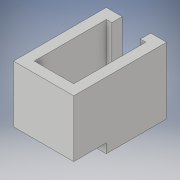
# Autodesk Inventor part: servo housing
Saved by Autodesk Inventor 2017 (Build 210142000, 142)
## iProperties
Created: 2017-01-19
Part Number: servo housing
Material: Generic
Document SubType Name: Modeling
Designer: Gabe Madonna
Density: 1 g/cm^3
Appearance: Default
Author: Gabe Madonna
Autodesk Inventor part; units mm, degrees
ref_plane "YZ Plane" through (0, 0, 0) normal (1, 0, 0) x (0, 1, 0)
ref_plane "XZ Plane" through (0, 0, 0) normal (0, 1, 0) x (-1, 0, 0)
ref_plane "XY Plane" through (0, 0, 0) normal (0, 0, 1) x (1, 0, 0)
sketch "Sketch1" plane through (0, 0, 0) normal (0, 1, 0) x (-1, 0, 0)
  line L0 (6.225, 11.375) -> (-6.225, 11.375)
  line L1 (-6.225, 11.375) -> (-6.225, -11.375)
  line L2 (-6.225, -11.375) -> (6.225, -11.375)
  line L3 (6.225, -11.375) -> (6.225, 11.375)
  line L4 (6.225, 11.375) -> (-6.225, -11.375) construction
  line L5 (-6.225, 11.375) -> (6.225, -11.375) construction
  line L6 (9.525, 14.675) -> (-9.525, 14.675)
  line L7 (-9.525, 14.675) -> (-9.525, -14.675)
  line L8 (-9.525, -14.675) -> (9.525, -14.675)
  line L9 (9.525, -14.675) -> (9.525, 14.675)
  point P0 (0, 0)
  dimension "d0" = 12.45
  dimension "d1" = 22.75
  dimension "d2" = 3.3
  constraints: 20 end point, 4 parallel, 2 midpoint, 2 perpendicular, 1 horizontal, 3 other
  measures "d0" distance of L2.end L1.end
  measures "d1" distance of L2.end L0.start
  measures "d2" distance between parallel lines of L3 L9
extrude "Extrusion1" add sketch "Sketch1" along normal blind 15
sketch "Sketch2" plane through (9.525, 0, -14.675) normal (0, 0, -1) x (-1, 0, 0)
  line L0 (14.025, 2.55) -> (5.025, 2.55)
  line L1 (5.025, 2.55) -> (5.025, 6.55)
  line L2 (14.025, 6.55) -> (14.025, 2.55)
  line L3 (3.3, 15) -> (15.75, 15) projected
  line L4 (5.025, 2.55) -> (14.025, 2.55)
  line L5 (14.025, 2.55) -> (14.025, 15)
  line L6 (14.025, 15) -> (5.025, 15)
  line L7 (5.025, 15) -> (5.025, 2.55)
  point P0 (9.525, 0)
  dimension "d7" = 9
  dimension "d8" = 4
  constraints: 14 end point, 3 parallel, 2 horizontal, 2 perpendicular, 1 point on line
  measures "d7" distance of L1.end L2.start
  measures "d8" distance of L2.start L0.start
extrude "Extrusion2" cut sketch "Sketch2" against normal up to next
sketch "Sketch3" plane through (0, 0, 0) normal (0, -1, 0) x (1, 0, 0)
  line L0 (-9.525, 14.675) -> (9.525, 14.675) projected
  line L1 (-9.525, -14.675) -> (-9.525, 14.675) projected
  line L2 (9.525, -14.675) -> (-9.525, -14.675) projected
  line L3 (9.525, 14.675) -> (9.525, -14.675) projected
  point P0 (0, 0)
extrude "Extrusion3" add sketch "Sketch3" along normal blind 3
sketch "Sketch4" plane through (0, -3, 0) normal (0, -1, 0) x (1, 0, 0)
  line L0 (6.225, 11.375) -> (6.225, -11.375) projected
  line L1 (6.225, -11.375) -> (-6.225, -11.375) projected
  line L2 (-6.225, -11.375) -> (-6.225, 11.375) projected
  line L3 (4.5, -11.375) -> (-4.5, -11.375) projected
  line L4 (0, -11.375) -> (0, -5.425)
  circle A0 centre (0, -5.425) radius 1
  point P0 (0, 0)
  dimension "d13" = 5.95
  dimension "d14" = 2
  constraints: 2 end point, 1 centre point, 1 coincident, 1 midpoint, 1 vertical
  measures "d13" distance of L4.start L4.end
  measures "d14" diameter of A0
extrude "Extrusion4" cut sketch "Sketch4" against normal up to next
sketch "Sketch5" plane through (0, -3, 0) normal (0, -1, 0) x (1, 0, 0)
  circle A0 centre (0, -5.425) radius 1 projected
  line L0 (-9.525, -14.675) -> (9.525, -14.675) projected
  line L1 (9.525, -14.675) -> (9.525, 4.375)
  line L2 (9.525, 4.375) -> (-9.525, 4.375)
  line L3 (-9.525, 4.375) -> (-9.525, -14.675)
  line L4 (-9.525, -14.675) -> (9.525, -14.675)
  line L5 (9.525, -14.675) -> (9.525, 4.375)
  point P0 (0, 0)
  dimension "d17" = 19.05
  constraints: 10 end point, 2 parallel, 1 horizontal, 1 perpendicular
  measures "d17" distance of L0.end L1.end
extrude "Extrusion5" add sketch "Sketch5" along normal blind 3
body "Solid1"
